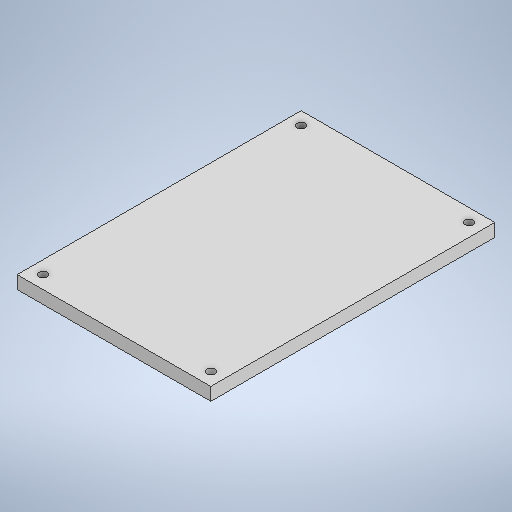
# Autodesk Inventor part: DAQ_HousingCover_V1
Saved by Autodesk Inventor 2025.2 (Build 292293000, 293)
## iProperties
Created: 2025-04-28
Part Number: DAQ_HousingCover_V1
Material: Generic
Document SubType Name: Modeling
Designer: limee
Density: 1 g/cm^3
Appearance: Default
Author: limee
Autodesk Inventor part; units mm, degrees
ref_plane "YZ Plane" through (0, 0, 0) normal (1, 0, 0) x (0, 1, 0)
ref_plane "XZ Plane" through (0, 0, 0) normal (0, 1, 0) x (-1, 0, 0)
ref_plane "XY Plane" through (0, 0, 0) normal (0, 0, 1) x (1, 0, 0)
sketch "Sketch1" plane through (0, 0, 0) normal (0, 1, 0) x (-1, 0, 0)
  line L0 (-37.5, 55) -> (37.5, 55)
  line L1 (37.5, 55) -> (37.5, -55)
  line L2 (37.5, -55) -> (-37.5, -55)
  line L3 (-37.5, -55) -> (-37.5, 55)
  line L4 (-37.5, 55) -> (37.5, -55) construction
  line L5 (37.5, 55) -> (-37.5, -55) construction
  point P0 (0, 0)
  dimension "d0" = 75
  dimension "d1" = 110
  constraints: 12 end point, 2 midpoint, 2 parallel, 1 horizontal, 1 perpendicular
  measures "d0" distance between parallel lines of L3 L1
  measures "d1" distance of L2.end L0.start
extrude "Extrusion1" add sketch "Sketch1" along normal blind 5
sketch "Sketch2" plane through (0, 5, 0) normal (0, 1, 0) x (1, 0, 0)
  line L0 (37.5, -55) -> (37.5, 55) projected
  line L1 (-37.5, -55) -> (37.5, -55) projected
  line L2 (37.5, 55) -> (-37.5, 55) projected
  line L3 (-37.5, 55) -> (-37.5, -55) projected
  point P0 (0, 0)
  point P1 (32.5, -50)
  point P2 (32.5, 50)
  point P3 (-32.5, 50)
  point P4 (-32.5, -50)
  dimension "HS" = 5
  dimension "d12" = 5
  dimension "d13" = 5
  dimension "d14" = 5
  constraints: 2 horizontal alignment, 2 vertical alignment
  measures "HS" distance from line of point (32.5, -50) L0
  measures "d12" distance from line of L1 point (-32.5, -50)
  measures "d13" distance from line of L2 point (-32.5, 50)
  measures "d14" distance from line of L3 point (-32.5, -50)
hole "Hole1" at (32.5, 5, 50) at (32.5, 5, -50) at (-32.5, 5, -50) at (-32.5, 5, 50) direction (0, -1, 0) diameter 3.2 depth 6
equation "\"d12\" = HS"
equation "\"d13\" = HS"
equation "\"d14\" = HS"
body "Solid1"
